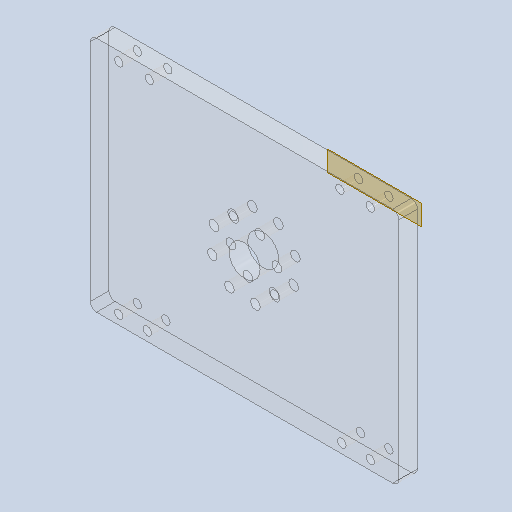
# Autodesk Inventor part: _pelvis
Saved by Autodesk Inventor 2024.3 (Build 283343000, 343)
## iProperties
Created: 2024-09-07
Part Number: _pelvis
Material: PMMA 플라스틱
Document SubType Name: Modeling
Designer: gretc
Density: 1.188 g/cm^3
Appearance: 폴리카보네이트 - 선명
Mass: 53.0622 g
Surface Area: 180.457 cm^2
Volume: 44.6651 cm^3
Author: gretc
Autodesk Inventor part; units mm, degrees
ref_plane "YZ Plane" through (0, 0, 0) normal (1, 0, 0) x (0, 1, 0)
ref_plane "XZ Plane" through (0, 0, 0) normal (0, 1, 0) x (-1, 0, 0)
ref_plane "XY Plane" through (0, 0, 0) normal (0, 0, 1) x (1, 0, 0)
ref_plane "작업 평면1" through (0, 0, 0) normal (0, 0, 1) x (1, 0, 0)
ref_plane "작업 평면2" through (0, 0, 0) normal (0, 0, 1) x (1, 0, 0)
sketch "스케치2" plane through (0, 0, 0) normal (0, 0, 1) x (1, 0, 0)
  circle A0 centre (-53.6, -73.63) radius 1.35 projected
  circle A1 centre (-62.8, -73.63) radius 1.35 projected
  line L0 (-72, -70.63) -> (-44.4, -70.63) projected
  line L1 (-72, -70.63) -> (-72, -76.63) projected
  line L2 (-72, -76.63) -> (-44.4, -76.63) projected
  line L3 (-44.4, -70.63) -> (-44.4, -76.63) projected
  circle A2 centre (18.4, -73.63) radius 1.35 projected
  circle A3 centre (9.2, -73.63) radius 1.35 projected
  line L4 (0, -70.63) -> (27.6, -70.63) projected
  line L5 (0, -70.63) -> (0, -76.63) projected
  line L6 (0, -76.63) -> (27.6, -76.63) projected
  line L7 (27.6, -70.63) -> (27.6, -76.63) projected
  circle A4 centre (18.4, -3) radius 1.35 projected
  circle A5 centre (8.5755, -3) radius 1.35 projected
  line L8 (0, 0) -> (27.6, 0) projected
  line L9 (0, 0) -> (0, -6) projected
  line L10 (0, -6) -> (27.6, -6) projected
  line L11 (27.6, 0) -> (27.6, -6) projected
  circle A6 centre (-62.8, -3) radius 1.35 projected
  circle A7 centre (-52.9755, -3) radius 1.35 projected
  line L12 (-44.4, 0) -> (-72, 0) projected
  line L13 (-72, 0) -> (-72, -6) projected
  line L14 (-44.4, -6) -> (-72, -6) projected
  line L15 (-44.4, 0) -> (-44.4, -6) projected
  line L16 (27.6, 0) -> (27.6, -76.63)
  line L17 (27.6, -76.63) -> (-72, -76.63)
  line L18 (-72, -76.63) -> (-72, 0)
  line L19 (-72, 0) -> (27.6, 0)
  point P0 (27.6, -70.63)
  point P1 (27.6, -6)
  constraints: 8 end point, 2 parallel, 1 perpendicular, 1 vertical
extrude "돌출1" add sketch "스케치2" along normal blind 6
sketch "스케치3" plane through (0, 0, 6) normal (0, 0, 1) x (1, 0, 0)
  line L0 (-72, -76.63) -> (27.6, -76.63) projected
  line L1 (27.6, 0) -> (-72, 0) projected
  line L2 (-72, -76.63) -> (-72, 0)
  line L3 (-72, 0) -> (-72, -42.4915)
  line L4 (-22.2, -76.63) -> (-22.2, 0)
  line L5 (-72, -38.315) -> (27.6, -38.315)
  circle A0 centre (-22.2, -38.315) radius 5
  point P0 (0, 0)
  dimension "d3" = 10
  constraints: 8 end point, 3 midpoint, 2 point on line, 1 centre point, 1 coincident, 1 perpendicular, 1 vertical
  measures "d3" diameter of A0
extrude "돌출2" cut sketch "스케치3" against normal blind 6 contours A0 L5 L4 | L4 L5 A0 | L5 A0 L4 | L4 A0 L5
sketch "스케치4" plane through (0, 0, 6) normal (0, 0, 1) x (1, 0, 0)
  circle A0 centre (-22.2, -38.315) radius 13.9 projected
  circle A1 centre (-25.6914, -27.8838) radius 1.25 projected
  circle A2 centre (-32.0448, -33.4078) radius 1.55 projected
  circle A3 centre (-17.2928, -28.4702) radius 1.25 projected
  circle A4 centre (-11.7688, -34.8236) radius 1.25 projected
  circle A5 centre (-12.3552, -43.2222) radius 1.25 projected
  circle A6 centre (-18.7086, -48.7462) radius 1.55 projected
  circle A7 centre (-27.1072, -48.1598) radius 1.55 projected
  circle A8 centre (-32.6312, -41.8064) radius 1.55 projected
  circle A9 centre (-25.6914, -27.8838) radius 1.55 projected
  circle A10 centre (-17.2928, -28.4702) radius 1.55 projected
  circle A11 centre (-11.7688, -34.8236) radius 1.55 projected
  circle A12 centre (-12.3552, -43.2222) radius 1.55 projected
  circle A13 centre (-32.6312, -41.8064) radius 1.25 projected
  circle A14 centre (-27.1072, -48.1598) radius 1.25 projected
  circle A15 centre (-18.7086, -48.7462) radius 1.25 projected
  circle A16 centre (-32.0448, -33.4078) radius 1.25 projected
  point P0 (0, 0)
extrude "돌출3" cut sketch "스케치4" against normal blind 6 contours A1 | A2 | A3 | A4 | A5 | A6 | A7 | A8 | A9 | A10 | A11 | A12 | A13 | A14 | A15 | A16
fillet "모깎기1" radius 2 4 edges at (-72, 0, 3) (27.6, 0, 3) (27.6, -76.63, 3) (-72, -76.63, 3)
